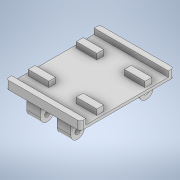
# Autodesk Inventor part: нижняя защелка пушки 2
Saved by Autodesk Inventor 2020.1 (Build 241239000, 239)
## iProperties
Created: 2022-04-03
Part Number: нижняя защелка пушки 2
Material: Типовые
Document SubType Name: Modeling
Designer: User
Density: 1 g/cm^3
Appearance: По умолчанию
Author: User
Autodesk Inventor part; units mm, degrees
ref_plane "YZ Plane" through (0, 0, 0) normal (1, 0, 0) x (0, 1, 0)
ref_plane "XZ Plane" through (0, 0, 0) normal (0, 1, 0) x (-1, 0, 0)
ref_plane "XY Plane" through (0, 0, 0) normal (0, 0, 1) x (1, 0, 0)
sketch "Эскиз1" plane through (0, 0, 0) normal (0, 1, 0) x (-1, 0, 0)
  line L0 (0, 0) -> (-27, 0)
  line L1 (-27, 0) -> (-27, 30)
  line L2 (-27, 30) -> (0, 30)
  line L3 (0, 30) -> (0, 0)
  dimension "d0" = 27
  dimension "d1" = 30
  constraints: 8 end point, 2 parallel, 1 horizontal, 1 perpendicular
  measures "d0" distance of L0.start L0.end
  measures "d1" distance of L0.end L1.end
extrude "Выдавливание1" add sketch "Эскиз1" along normal blind 2
sketch "Эскиз2" plane through (0, 2, 0) normal (0, 1, 0) x (1, 0, 0)
  line L0 (0, 0) -> (0, -30) projected
  line L1 (0, 0) -> (25, 0)
  line L2 (25, 0) -> (25, -20)
  line L3 (25, -20) -> (0, -20)
  line L4 (0, -20) -> (0, 0)
  line L5 (25, -20) -> (10, -20)
  line L6 (10, -20) -> (10, -15)
  line L7 (10, -15) -> (25, -15)
  line L8 (25, -15) -> (25, -20)
  dimension "d4" = 25
  dimension "d5" = 20
  dimension "d6" = 5
  dimension "d7" = 15
  constraints: 16 end point, 4 parallel, 2 horizontal, 2 perpendicular
  measures "d4" distance of L2.end L3.end
  measures "d5" distance of L1.end L2.end
  measures "d6" distance of L5.end L6.end
  measures "d7" distance of L6.end L7.end
extrude "Выдавливание2" add sketch "Эскиз2" along normal blind 4 contours L6 L7 L2 L3
sketch "Эскиз3" plane through (0, 0, 0) normal (0, -1, 0) x (1, 0, 0)
  line L0 (6, 30) -> (16, 30)
  line L1 (16, 30) -> (16, 20)
  line L2 (16, 20) -> (6, 20)
  line L3 (6, 20) -> (6, 30)
  line L4 (27, 0) -> (0, 0) projected
  line L5 (0, 0) -> (0, 30) projected
  dimension "d10" = 20
  dimension "d11" = 10
  dimension "d12" = 10
  dimension "d13" = 6
  constraints: 8 end point, 2 parallel, 1 horizontal, 1 perpendicular
  measures "d10" distance between parallel lines of L2 L4
  measures "d11" distance of L0.end L1.end
  measures "d12" distance of L0.start L0.end
  measures "d13" distance from line of L5 L0.start
extrude "Выдавливание3" add sketch "Эскиз3" along normal blind 15
sketch "Эскиз4" plane through (16, 0, 30) normal (1, 0, 0) x (0, 0, -1)
  line L0 (0, 0) -> (0, -15) projected
  line L1 (10, -15) -> (0, -15) projected
  circle A0 centre (5, -10) radius 2
  point P0 (30, 0)
  point P1 (0, -10)
  point P2 (5, -15)
  dimension "d16" = 5
  dimension "d17" = 4
  constraints: 1 centre point, 1 midpoint, 1 point on line
  measures "d16" distance from line of L1 point (0, -10)
  measures "d17" diameter of A0
extrude "Выдавливание4" cut sketch "Эскиз4" against normal blind 10
fillet "Сопряжение1" radius 5 2 edges at (11, -15, 30) (11, -15, 20)
sketch "Эскиз5" plane through (0, 2, 30) normal (0, 0, 1) x (1, 0, 0)
  line L0 (0, -2) -> (6, -2) projected
  line L1 (27, -2) -> (27, 0) projected
  line L2 (0, -2) -> (27, -2)
  line L3 (27, -2) -> (27, 0)
  line L4 (27, 0) -> (0, 0)
  line L5 (0, 0) -> (0, -2)
  constraints: 8 end point, 2 parallel, 1 horizontal, 1 perpendicular
extrude "Выдавливание5" add sketch "Эскиз5" along normal blind 4
sketch "Эскиз6" plane through (0, 2, 0) normal (0, 1, 0) x (1, 0, 0)
  line L0 (27, -34) -> (0, -34) projected
  line L1 (0, 0) -> (0, -34) projected
  line L2 (27, -34) -> (0, -34)
  line L3 (0, -34) -> (0, -30)
  line L4 (0, -30) -> (27, -30)
  line L5 (27, -30) -> (27, -34)
  dimension "d23" = 4
  constraints: 8 end point, 2 parallel, 1 horizontal, 1 perpendicular, 1 point on line
  measures "d23" distance between parallel lines of L0 L4
extrude "Выдавливание6" add sketch "Эскиз6" along normal blind 4
mirror "Зеркальное отражение1" about plane through (0, 0, 0) normal (-1, 0, 0)
mirror "Зеркальное отражение2" about plane through (27, 0, 0) normal (0, 0, -1)
fillet "Сопряжение2" radius 2 4 edges at (27, 3, 34) (27, 3, -34) (-27, 3, -34) (-27, 3, 34)
